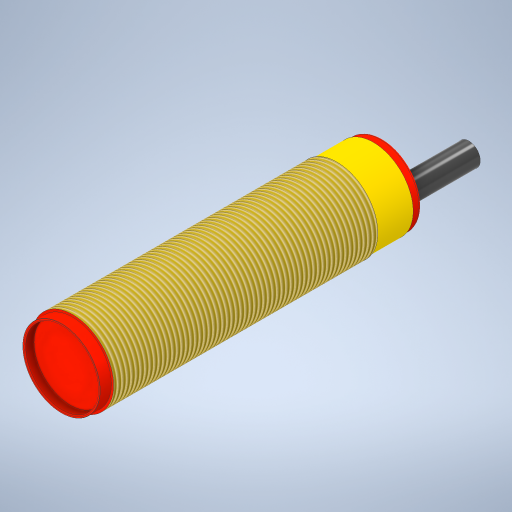
# Autodesk Inventor part: 2309HCMUTE-CDT23-CB_E3F-DS30C4
Saved by Autodesk Inventor 2023 (Build 270158000, 158)
## iProperties
Created: 2023-10-11
Part Number: 2309HCMUTE-CDT23-CB_E3F-DS30C4
Material: PVC-Piping
Document SubType Name: Modeling
Designer: havie
Density: 1.4 g/cm^3
Appearance: Smooth - White
Author: havie
Autodesk Inventor part; units mm, degrees
ref_plane "YZ Plane" through (0, 0, 0) normal (1, 0, 0) x (0, 1, 0)
ref_plane "XZ Plane" through (0, 0, 0) normal (0, 1, 0) x (-1, 0, 0)
ref_plane "XY Plane" through (0, 0, 0) normal (0, 0, 1) x (1, 0, 0)
sketch "Sketch1" plane through (0, 0, 0) normal (0, 1, 0) x (-1, 0, 0)
  circle A0 centre (0, 0) radius 9
  dimension "d0" = 18
  constraints: 1 centre point, 1 coincident
  measures "d0" diameter of A0
extrude "Extrusion1" add sketch "Sketch1" along normal mid plane 58
thread "Thread1"
sketch "Sketch2" plane through (0, -29, 0) normal (0, -1, 0) x (1, 0, 0)
  circle A0 centre (0, 0) radius 8.5
  dimension "d13" = 17
  constraints: 1 centre point, 1 coincident
  measures "d13" diameter of A0
extrude "Extrusion2" add sketch "Sketch2" along normal blind 2.5
sketch "Sketch3" plane through (0, -31.5, 0) normal (0, -1, 0) x (1, 0, 0)
  circle A0 centre (0, 0) radius 8
  circle A1 centre (0, 0) radius 8.5 projected
  dimension "d14" = 0.5
  constraints: 1 centre point, 1 coincident
  measures "d14" radial gap between concentric circles of A1 A0
extrude "Extrusion3" cut sketch "Sketch3" against normal blind 2 contours A0
fillet "Fillet1" radius 0.2 1 edges at (-8, -31.5, 0)
fillet "Fillet2" radius 0.05 1 edges at (-8.5, -31.5, 0)
sketch "Sketch4" plane through (0, 29, 0) normal (0, 1, 0) x (1, 0, 0)
  circle A0 centre (0, 0) radius 8.75
  dimension "d15" = 17.5
  constraints: 1 centre point, 1 coincident
  measures "d15" diameter of A0
extrude "Extrusion4" add sketch "Sketch4" along normal blind 8
sketch "Sketch5" plane through (0, 37, 0) normal (0, 1, 0) x (1, 0, 0)
  circle A0 centre (0, 0) radius 8.55
  circle A1 centre (0, 0) radius 8.75 projected
  dimension "d18" = 0.2
  constraints: 1 centre point, 1 coincident
  measures "d18" radial gap between concentric circles of A0 A1
extrude "Extrusion5" add sketch "Sketch5" along normal blind 2 contours A0
fillet "Fillet3" radius 0.5 1 edges at (-8.55, 39, 0)
sketch "Sketch6" plane through (0, 39, 0) normal (0, 1, 0) x (1, 0, 0)
  circle A0 centre (4, 0) radius 2.5
  point P0 (0, 0)
  dimension "d22" = 5
  dimension "d23" = 4
  constraints: 1 centre point, 1 horizontal alignment
  measures "d22" diameter of A0
  measures "d23" distance of point (0, 0) A0.centre
sketch3d "3D Sketch1"
  line L0 (4, 39, 0) -> (4, 54, 0)
  dimension "d26" = 15
sweep "Sweep2" add profiles "Sketch6" path "3D Sketch1"
sketch "Sketch7" plane through (0, 39, 0) normal (0, 1, 0) x (1, 0, 0)
  circle A0 centre (-3, -3) radius 2
  circle A1 centre (-3, -3) radius 1.45
  line L0 (-4.4283, -3.25) -> (-1.5717, -3.25)
  line L1 (-4.4283, -2.75) -> (-1.5717, -2.75)
  point P0 (0, 0)
  dimension "d29" = 4
  dimension "d30" = 3
  dimension "d31" = 3
  dimension "d32" = 2.9
  dimension "d33" = 0.5
  dimension "d34" = 0.25
  constraints: 4 end point, 4 point on circle, 2 centre point, 1 coincident, 1 horizontal, 1 parallel
  measures "d29" diameter of A0
  measures "d30" horizontal distance of point (0, 0) A0.centre
  measures "d31" horizontal distance of point (0, 0) A0.centre
  measures "d32" diameter of A1
  measures "d33" distance between parallel lines of L1 L0
  measures "d34" distance from line of A0.centre L0
extrude "Extrusion6" cut sketch "Sketch7" against normal blind 0.5
extrude "Extrusion7" cut sketch "Sketch7" against normal blind 0.3 contours A1 L0 L1
sketch "Sketch8" plane through (0, 39, 0) normal (0, 1, 0) x (1, 0, 0)
  circle A0 centre (-3, 4) radius 0.75
  point P0 (0, 0)
  dimension "d39" = 1.5
  dimension "d40" = 4
  dimension "d41" = 3
  constraints: 1 centre point
  measures "d39" diameter of A0
  measures "d40" vertical distance of point (0, 0) A0.centre
  measures "d41" horizontal distance of point (0, 0) A0.centre
extrude "Extrusion8" add sketch "Sketch8" along normal blind 1
fillet "Fillet4" radius 0.75 1 edges at (-3.75, 40, -4)
sketch "Sketch9" plane through (0, -29.5, 0) normal (0, -1, 0) x (1, 0, 0)
  line L0 (1.5, 5) -> (-1.5, 5)
  line L1 (-1.5, 5) -> (-1.5, 1)
  line L2 (-1.5, 1) -> (1.5, 1)
  line L3 (1.5, 1) -> (1.5, 5)
  line L4 (1.5, -1) -> (-1.5, -1)
  line L5 (-1.5, -1) -> (-1.5, -5)
  line L6 (-1.5, -5) -> (1.5, -5)
  line L7 (1.5, -5) -> (1.5, -1)
  point P0 (0, 0)
  point P1 (0, 1)
  dimension "d45" = 4
  dimension "d46" = 4
  dimension "d47" = 3
  dimension "d48" = 2
  dimension "d49" = 1
  constraints: 16 end point, 4 parallel, 3 vertical alignment, 2 horizontal, 2 perpendicular, 2 point on line, 1 midpoint
  measures "d45" distance of L2.end L0.start
  measures "d46" distance of L6.end L4.start
  measures "d47" distance of L1.end L2.end
  measures "d48" distance between parallel lines of L4 L2
  measures "d49" distance from line of L4 point (0, 0)
sketch "Sketch10" plane through (0, 0, 0) normal (1, 0, 0) x (0, 1, 0)
  line L0 (-29.5, -5) -> (-29.5, -1) projected
  line L1 (-29.5, 1) -> (-29.5, 5) projected
  spline S0 degree 2 poles (-29.5, -1) (-31.582, -1.7446) (-29.5, -5) knots 0 0 0 1 1 1
  spline S1 degree 2 poles (-29.5, 1) (-31.5, 3) (-29.5, 5) knots 0 0 0 1 1 1
  line L2 (-29.5, -8) -> (-29.5, 8) projected
  point P0 (0, 0)
  point P1 (-30.5, -2)
  point P2 (-30.5, 3)
  dimension "d50" = 5
  dimension "d51" = 1
  dimension "d52" = 6
  constraints: 1 vertical alignment, 6 other
  measures "d50" distance of point (-30.5, 3) point (-30.5, -2)
  measures "d51" distance from line of L2 point (-30.5, -2)
  measures "d52" vertical distance of L2.start point (-30.5, -2)
body "Solid1"
body "Srf1"
body "Srf2"
